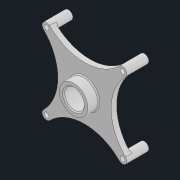
# Autodesk Inventor part: scara-base12
Saved by Autodesk Inventor 2022 (Build 260153000, 153)
## iProperties
Created: 2021-10-28
Part Number: scara-base12
Material: 一般
Document SubType Name: Modeling
Designer: Yuta Kage
Density: 1 g/cm^3
Appearance: 既定
Author: Yuta Kage
Autodesk Inventor part; units mm, degrees
ref_plane "YZ Plane" through (0, 0, 0) normal (1, 0, 0) x (0, 1, 0)
ref_plane "XZ Plane" through (0, 0, 0) normal (0, 1, 0) x (-1, 0, 0)
ref_plane "XY Plane" through (0, 0, 0) normal (0, 0, 1) x (1, 0, 0)
sketch "スケッチ1" plane through (0, 0, 0) normal (0, 0, 1) x (1, 0, 0)
  circle A0 centre (0, 0) radius 49 construction
  circle A1 centre (-34.6482, 34.6482) radius 4
  circle A2 centre (-34.6482, -34.6482) radius 4
  circle A3 centre (34.6482, -34.6482) radius 4
  circle A4 centre (34.6482, 34.6482) radius 4
  circle A5 centre (0, 69.2965) radius 45
  circle A6 centre (-69.2965, 0) radius 45
  circle A7 centre (0, -69.2965) radius 45
  circle A8 centre (69.2965, 0) radius 45
  line L0 (-38.6482, -38.6482) -> (38.6482, -38.6482)
  line L1 (38.6482, -38.6482) -> (38.6482, 38.6482)
  line L2 (38.6482, 38.6482) -> (-38.6482, 38.6482)
  line L3 (-38.6482, 38.6482) -> (-38.6482, -38.6482)
  line L4 (-38.6482, -38.6482) -> (38.6482, 38.6482) construction
  line L5 (38.6482, -38.6482) -> (-38.6482, 38.6482) construction
  line L6 (0, 69.2965) -> (-69.2965, 0)
  circle A9 centre (0, 0) radius 13
  point P0 (0, 24.2965)
  point P1 (-24.2965, 0)
  point P2 (0, -24.2965)
  point P3 (24.2965, 0)
  point P4 (37.4767, -31.8198)
  point P5 (37.4767, 31.8198)
  point P6 (31.8198, 37.4767)
  point P7 (-31.8198, 37.4767)
  point P8 (-37.4767, 31.8198)
  point P9 (-37.4767, -31.8198)
  point P10 (-31.8198, -37.4767)
  point P11 (31.8198, -37.4767)
  dimension "d0" = 98
  dimension "d1" = 8
  dimension "d4" = 360
  dimension "d9" = 360
  dimension "d27" = 26
  constraints: 14 end point, 5 centre point, 3 midpoint, 2 coincident, 2 parallel, 2 tangent, 1 horizontal, 1 horizontal alignment, 1 perpendicular, 1 vertical alignment, 39 other
  measures "d1" diameter of A1
  measures "d27" diameter of A9
extrude "押し出し1" add sketch "スケッチ1" along normal blind 5 contours A1 L6 | A1 A5 A4 A8 A3 A7 A2 A6 | L6 A1 | A4 | A2 | A3 | A9
extrude "押し出し4" add sketch "スケッチ1" against normal blind 15 contours A1 L6 | L6 A1 | A4 | A2 | A3
sketch "スケッチ6" plane through (-34.6482, -34.6482, -15) normal (0, 0, -1) x (-1, 0, 0)
  circle A0 centre (-69.2965, 0) radius 4 projected
  circle A1 centre (0, 0) radius 4 projected
  circle A2 centre (0, 69.2965) radius 4 projected
  circle A3 centre (-69.2965, 69.2965) radius 4 projected
  point P0 (-34.6482, 34.6482)
hole "穴1" at (-34.6482, -34.6482, -15) at (34.6482, -34.6482, -15) at (-34.6482, 34.6482, -15) at (34.6482, 34.6482, -15) direction (0, 0, 1) diameter 4.5 end through all clearance for "Flat Head Machine Screw" size "M4" standard "Ansi Metric M Profile"
sketch "スケッチ7" plane through (0, 0, 5) normal (0, 0, -1) x (-1, 0, 0)
  circle A0 centre (0, 0) radius 13
  dimension "d38" = 26
  constraints: 1 centre point, 1 coincident
  measures "d38" diameter of A0
extrude "押し出し6" add sketch "スケッチ7" against normal blind 10
sketch "スケッチ8" plane through (0, 0, 15) normal (0, 0, 1) x (1, 0, 0)
  circle A0 centre (0, 0) radius 9
  dimension "d41" = 18
  constraints: 1 centre point, 1 coincident
  measures "d41" diameter of A0
extrude "押し出し7" cut sketch "スケッチ8" against normal through all
chamfer "面取り1" distance 1 angle 45 2 edges at (-9, 0, 15) (13, 0, 5)
chamfer "面取り2" distance 1 angle 45 6 edges at (31.8198, -31.8198, 0) (-33.1175, -30.9527, 0) (-30.9527, -36.179, 0) (-30.9527, 36.179, 0) (-33.1175, 30.9527, 0) (31.8198, 31.8198, 0)
chamfer "面取り4" distance 1 angle 45 1 edges at (-9, 0, 0)
ref_plane "作業平面2" through (0, 0, 2.5) normal (0, 0, 1) x (1, 0, 0)
